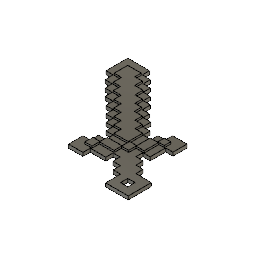
minecraft sword v1 (Autodesk Fusion 360 design; units mm, degrees)
Autodesk Fusion 360 part; units mm, degrees
sketch "sword" plane through (0, 0, 0) normal (0, 0, 1) x (1, 0, 0)
  line L0 (-55, 55) -> (45, 55)
  line L1 (45, 55) -> (45, -15)
  line L2 (45, -15) -> (-55, -15)
  line L3 (-55, -15) -> (-55, 55)
  line L4 (-30.5, 51.5) -> (-18.5, 51.5)
  line L5 (-18.5, 51.5) -> (-18.5, 47.5)
  line L6 (-18.5, 47.5) -> (-14, 47.5)
  line L7 (-14, 47.5) -> (-14, 43.5)
  line L8 (-14, 43.5) -> (-10, 43.5)
  line L9 (-10, 43.5) -> (-10, 39.5)
  line L10 (-10, 39.5) -> (-6, 39.5)
  line L11 (-6, 39.5) -> (-6, 35.5)
  line L12 (-6, 35.5) -> (-2, 35.5)
  line L13 (-2, 35.5) -> (-2, 31)
  line L14 (-2, 31) -> (2, 31)
  line L15 (2, 31) -> (2, 27.5)
  line L16 (2, 27.5) -> (6.2436, 27.5)
  line L17 (6.2436, 27.5) -> (6.2436, 23)
  line L18 (6.2436, 23) -> (10.2565, 23)
  line L19 (10.2565, 23) -> (10.2565, 19.2336)
  line L20 (10.2565, 19.2336) -> (14.5, 19.2336)
  line L21 (14.5, 19.2336) -> (14.5, 23)
  line L22 (14.5, 23) -> (18.5, 23)
  line L23 (18.5, 23) -> (18.5, 27)
  line L24 (18.5, 27) -> (26.5, 27)
  line L25 (26.5, 27) -> (26.5, 19.2336)
  line L26 (26.5, 19.2336) -> (22.5, 19.2336)
  line L27 (22.5, 19.2336) -> (22.5, 10.7788)
  line L28 (22.5, 10.7788) -> (18.5, 10.7788)
  line L29 (18.5, 10.7788) -> (18.5, 7)
  line L30 (18.5, 7) -> (22.5, 7)
  line L31 (22.5, 7) -> (22.5, 3)
  line L32 (22.5, 3) -> (26.5, 3)
  line L33 (26.5, 3) -> (26.5, -1)
  line L34 (26.5, -1) -> (35, -1)
  line L35 (35, -1) -> (35, -13.7276)
  line L36 (35, -13.7276) -> (22.5, -13.7276)
  line L37 (22.5, -13.7276) -> (22.5, -5.5)
  line L38 (22.5, -5.5) -> (18.5, -5.5)
  line L39 (18.5, -5.5) -> (18.5, -1.5)
  line L40 (18.5, -1.5) -> (14.2693, -1.5)
  line L41 (14.2693, -1.5) -> (14.2693, 2.5)
  line L42 (14.2693, 2.5) -> (10.5, 2.5)
  line L43 (10.5, 2.5) -> (10.5, -1.5)
  line L44 (10.5, -1.5) -> (2, -1.5)
  line L45 (2, -1.5) -> (2, -5.5)
  line L46 (2, -5.5) -> (-6, -5.5)
  line L47 (-6, -5.5) -> (-6, 2.5)
  line L48 (-6, 2.5) -> (-2, 2.5)
  line L49 (-2, 2.5) -> (-2, 7)
  line L50 (-2, 7) -> (2, 7)
  line L51 (2, 7) -> (2, 11)
  line L52 (2, 11) -> (-2, 11)
  line L53 (-2, 11) -> (-2, 15)
  line L54 (-2, 15) -> (-6, 15)
  line L55 (-6, 15) -> (-6, 19)
  line L56 (-6, 19) -> (-10, 19)
  line L57 (-10, 19) -> (-10, 23)
  line L58 (-10, 23) -> (-14, 23)
  line L59 (-14, 23) -> (-14, 27)
  line L60 (-14, 27) -> (-18.5, 27)
  line L61 (-18.5, 27) -> (-18.5, 31)
  line L62 (-18.5, 31) -> (-22.5, 31)
  line L63 (-22.5, 31) -> (-22.5, 35)
  line L64 (-22.5, 35) -> (-26.5, 35)
  line L65 (-26.5, 35) -> (-26.5, 39.5)
  line L66 (-26.5, 39.5) -> (-30.5, 39.5)
  line L67 (-30.5, 39.5) -> (-30.5, 51.5)
  line L68 (26.5788, -5.5391) -> (30.5, -5.5391)
  line L69 (30.5, -5.5391) -> (30.5, -9.5)
  line L70 (30.5, -9.5) -> (26.5788, -9.5)
  line L71 (26.5788, -9.5) -> (26.5788, -5.5391)
  line L72 (-26, 47) -> (-18.632, 47)
  line L73 (-18.632, 47) -> (-18.632, 43.5639)
  line L74 (-18.632, 43.5639) -> (-14.5387, 43.5639)
  line L75 (-14.5387, 43.5639) -> (-14.5387, 39.3879)
  line L76 (-14.5387, 39.3879) -> (-10, 39.3879)
  line L77 (-10, 39.3879) -> (-10, 35)
  line L78 (-10, 35) -> (-6, 35)
  line L79 (-6, 35) -> (-6, 31)
  line L80 (-6, 31) -> (-2.3828, 31)
  line L81 (-2.3828, 31) -> (-2.3828, 27)
  line L82 (-2.3828, 27) -> (2, 27)
  line L83 (2, 27) -> (2, 23)
  line L84 (2, 23) -> (6, 23)
  line L85 (6, 23) -> (6, 19)
  line L86 (6, 19) -> (10.2565, 19)
  line L87 (10.2565, 19) -> (10.2565, 11)
  line L88 (10.2565, 11) -> (2.4134, 11)
  line L89 (2.4134, 11) -> (2.4134, 15)
  line L90 (2.4134, 15) -> (-1.6386, 15)
  line L91 (-1.6386, 15) -> (-1.6386, 19)
  line L92 (-1.6386, 19) -> (-5.5665, 19)
  line L93 (-5.5665, 19) -> (-5.5665, 23)
  line L94 (-5.5665, 23) -> (-9.6185, 23)
  line L95 (-9.6185, 23) -> (-9.6185, 27)
  line L96 (-9.6185, 27) -> (-13.6291, 27)
  line L97 (-13.6291, 27) -> (-13.6291, 31)
  line L98 (-13.6291, 31) -> (-18, 31)
  line L99 (-18, 31) -> (-18, 35)
  line L100 (-18, 35) -> (-22, 35)
  line L101 (-22, 35) -> (-22, 39.5533)
  line L102 (-22, 39.5533) -> (-26, 39.5533)
  line L103 (-26, 39.5533) -> (-26, 47)
  line L104 (18.4708, 22.5599) -> (22, 22.5599)
  line L105 (22, 22.5599) -> (22, 19)
  line L106 (22, 19) -> (19, 19)
  line L107 (19, 19) -> (19, 11)
  line L108 (19, 11) -> (14.5279, 11)
  line L109 (14.5279, 11) -> (14.5279, 7)
  line L110 (14.5279, 7) -> (10.5586, 7)
  line L111 (10.5586, 7) -> (10.5586, 3)
  line L112 (10.5586, 3) -> (2.4547, 3)
  line L113 (2.4547, 3) -> (2.4547, -1)
  line L114 (2.4547, -1) -> (-1.4732, -1)
  line L115 (-1.4732, -1) -> (-1.4732, 3.4164)
  line L116 (-1.4732, 3.4164) -> (2.4547, 3.4164)
  line L117 (2.4547, 3.4164) -> (2.4547, 7.3444)
  line L118 (2.4547, 7.3444) -> (10.5586, 7.3444)
  line L119 (10.5586, 7.3444) -> (10.5586, 11.4377)
  line L120 (10.5586, 11.4377) -> (14.5279, 11.4377)
  line L121 (14.5279, 11.4377) -> (14.5, 18.756)
  line L122 (14.5, 18.756) -> (18.4708, 18.7711)
  line L123 (18.4708, 18.7711) -> (18.4708, 22.5599)
  constraint horizontal L0
  constraint vertical L1
  constraint horizontal L2
  constraint vertical L3
  constraint parallel L2 L4
  constraint perpendicular L4 L5
  constraint perpendicular L5 L6
  constraint perpendicular L4 L7
  constraint perpendicular L7 L8
  constraint perpendicular L4 L9
  constraint perpendicular L7 L10
  constraint perpendicular L4 L11
  constraint perpendicular L7 L12
  constraint perpendicular L4 L13
  constraint perpendicular L13 L14
  constraint perpendicular L4 L15
  constraint perpendicular L13 L16
  constraint perpendicular L16 L17
  constraint perpendicular L17 L18
  constraint perpendicular L18 L19
  constraint perpendicular L17 L20
  constraint perpendicular L18 L21
  constraint perpendicular L21 L22
  constraint perpendicular L18 L23
  constraint perpendicular L23 L24
  constraint perpendicular L18 L25
  constraint perpendicular L23 L26
  constraint perpendicular L26 L27
  constraint perpendicular L23 L28
  constraint perpendicular L26 L29
  constraint perpendicular L23 L30
  constraint perpendicular L26 L31
  constraint perpendicular L23 L32
  constraint perpendicular L32 L33
  constraint perpendicular L23 L34
  constraint perpendicular L32 L35
  constraint perpendicular L35 L36
  constraint perpendicular L36 L37
  constraint perpendicular L35 L38
  constraint perpendicular L36 L39
  constraint perpendicular L35 L40
  constraint perpendicular L36 L41
  constraint perpendicular L35 L42
  constraint perpendicular L36 L43
  constraint perpendicular L43 L44
  constraint perpendicular L36 L45
  constraint perpendicular L43 L46
  constraint perpendicular L36 L47
  constraint perpendicular L47 L48
  constraint perpendicular L48 L49
  constraint perpendicular L49 L50
  constraint perpendicular L50 L51
  constraint perpendicular L49 L52
  constraint perpendicular L52 L53
  constraint perpendicular L53 L54
  constraint perpendicular L54 L55
  constraint perpendicular L55 L56
  constraint perpendicular L56 L57
  constraint perpendicular L55 L58
  constraint perpendicular L58 L59
  constraint perpendicular L55 L60
  constraint perpendicular L60 L61
  constraint perpendicular L61 L62
  constraint perpendicular L62 L63
  constraint perpendicular L61 L64
  constraint perpendicular L64 L65
  constraint perpendicular L65 L66
  constraint perpendicular L4 L67
  constraint parallel L66 L68
  constraint perpendicular L66 L69
  constraint perpendicular L69 L70
  constraint perpendicular L68 L71
  constraint horizontal L72
  constraint perpendicular L72 L73
  constraint perpendicular L73 L74
  constraint perpendicular L74 L75
  constraint perpendicular L75 L76
  constraint perpendicular L76 L77
  constraint perpendicular L75 L78
  constraint perpendicular L78 L79
  constraint perpendicular L79 L80
  constraint perpendicular L80 L81
  constraint perpendicular L79 L82
  constraint perpendicular L80 L83
  constraint perpendicular L79 L84
  constraint perpendicular L80 L85
  constraint perpendicular L19 L86
  constraint perpendicular L86 L87
  constraint perpendicular L19 L88
  constraint perpendicular L86 L89
  constraint perpendicular L89 L90
  constraint perpendicular L86 L91
  constraint perpendicular L55 L92
  constraint perpendicular L56 L93
  constraint perpendicular L93 L94
  constraint perpendicular L52 L95
  constraint perpendicular L95 L96
  constraint perpendicular L52 L97
  constraint perpendicular L61 L98
  constraint perpendicular L62 L99
  constraint perpendicular L61 L100
  constraint perpendicular L100 L101
  constraint perpendicular L65 L102
  constraint perpendicular L72 L103
  constraint horizontal L104
  constraint perpendicular L104 L105
  constraint perpendicular L105 L106
  constraint perpendicular L106 L107
  constraint perpendicular L105 L108
  constraint perpendicular L108 L109
  constraint perpendicular L105 L110
  constraint perpendicular L110 L111
  constraint perpendicular L105 L112
  constraint perpendicular L110 L113
  constraint perpendicular L113 L114
  constraint perpendicular L110 L115
  constraint perpendicular L113 L116
  constraint perpendicular L116 L117
  constraint perpendicular L113 L118
  constraint perpendicular L116 L119
  constraint perpendicular L113 L120
  constraint perpendicular L121 L122
  constraint perpendicular L104 L123
extrude "Extrude1" add sketch "sword" along normal blind 3 contours L72 L73 L74 L75 L76 L77 L78 L79 L80 L81 L82 L83 L84 L85 L86 L87 L88 L89 L90 L91 L92 L93 L94 L95 L96 L97 L98 L99 L100 L101 L102 L103 makes body 1
extrude "Extrude2" add sketch "sword" along normal blind 3 separate body contours L104 L105 L106 L107 L108 L109 L110 L111 L112 L113 L114 L115 L116 L117 L118 L119 L120 L121 L122 L123 makes body 2
extrude "Extrude3" add sketch "sword" along normal blind 2 contours L4 L5 L6 L7 L8 L9 L10 L11 L12 L13 L14 L15 L16 L17 L18 L19 L20 L21 L22 L23 L24 L25 L26 L27 L28 L29 L30 L31 L32 L33 L34 L35 L36 L37 L38 L39 L40 L41 L42 L43 L44 L45 L46 L47 L48 L49 L50 L51 L52 L53 L54 L55 L56 L57 L58 L59 L60 L61 L62 L63 L64 L65 L66 L67 bodies 1 2
named bodies: "sword"
